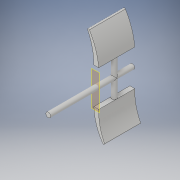
# Autodesk Inventor part: wet_proj_aandrijstang_2
Saved by Autodesk Inventor 2019.3 (Build 233278000, 278)
## iProperties
Created: 2020-03-03
Part Number: wet_proj_aandrijstang_2
Material: Generic
Document SubType Name: Modeling
Designer: Trial
Density: 1 g/cm^3
Appearance: Default
Author: Trial
Autodesk Inventor part; units mm, degrees
ref_plane "YZ Plane" through (0, 0, 0) normal (1, 0, 0) x (0, 1, 0)
ref_plane "XZ Plane" through (0, 0, 0) normal (0, 1, 0) x (-1, 0, 0)
ref_plane "XY Plane" through (0, 0, 0) normal (0, 0, 1) x (1, 0, 0)
sketch "Sketch1" plane through (0, 0, 0) normal (0, 0, 1) x (1, 0, 0)
  circle A0 centre (0, 0) radius 5
  dimension "d0" = 10
  constraints: 1 centre point, 1 coincident
  measures "d0" diameter of A0
extrude "Extrusion1" add sketch "Sketch1" against normal blind 175
ref_plane "Work Plane1" through (0, 0, -100) normal (0, 0, 1) x (1, 0, 0)
sketch "Sketch2" plane through (0, 0, 0) normal (0, 1, 0) x (-1, 0, 0)
  circle A0 centre (0, -137.5) radius 5
  line L0 (-5, -175) -> (5, -175) projected
  point P0 (0, 0)
  dimension "d4" = 10
  dimension "d5" = 37.5
  constraints: 1 centre point
  measures "d4" diameter of A0
  measures "d5" distance from line of L0 A0.centre
extrude "Extrusion2" add sketch "Sketch2" along normal mid plane 75
sketch "Sketch5" plane through (0, 0, -100) normal (0, 0, 1) x (1, 0, 0)
  line L0 (5, 37.5) -> (-5, 37.5) projected
  arc A0 (-5, 37.5) -> (-18.5426, 95.9905) centre (-137.4066, 37.6564) ccw
  arc A1 (5, 37.5) -> (-14.4042, 96.255) centre (-129.1845, 25.7664) ccw
  arc A2 (-14.4042, 96.255) -> (-18.5426, 95.9905) centre (-16.4034, 95.0273) ccw
  line L1 (-5, -37.5) -> (5, -37.5) projected
  arc A3 (5, -37.5) -> (17.351, -93.4908) centre (120.393, -41.4031) ccw
  arc A4 (-5, -37.5) -> (13.2332, -94.5364) centre (105.5133, -33.604) ccw
  line L2 (5, -37.5) -> (-5, -37.5)
  line L3 (5, 37.5) -> (-5, 37.5)
  arc A5 (13.2332, -94.5364) -> (17.351, -93.4908) centre (15.1102, -93.297) ccw
  point P0 (0, 0)
  constraints: 12 point on circle, 6 centre point, 4 end point, 2 tangent, 1 collinear, 1 horizontal
extrude "Extrusion4" add sketch "Sketch5" against normal blind 75
body "Solid1"
